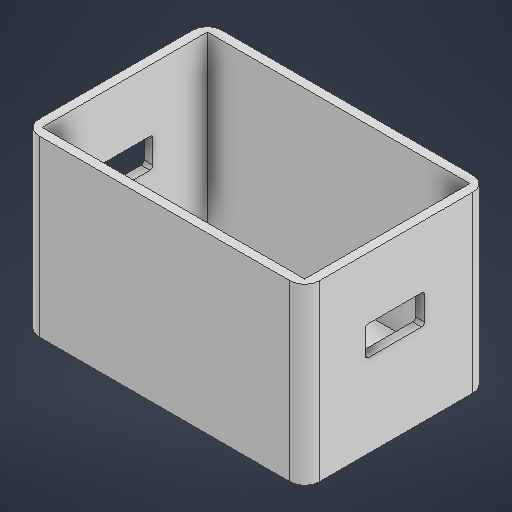
# Autodesk Inventor part: bottom
Saved by Autodesk Inventor 2026.1 (Build 301233020, 233B)
## iProperties
Created: 2025-11-06
Part Number: bottom
Material: Generisch
Document SubType Name: Modeling
Designer: sarae
Density: 1 g/cm^3
Appearance: Vorgabe
Author: sarae
Autodesk Inventor part; units mm, degrees
ref_plane "YZ Plane" through (0, 0, 0) normal (1, 0, 0) x (0, 1, 0)
ref_plane "XZ Plane" through (0, 0, 0) normal (0, 1, 0) x (-1, 0, 0)
ref_plane "XY Plane" through (0, 0, 0) normal (0, 0, 1) x (1, 0, 0)
sketch "Skizze1" plane through (0, 0, 0) normal (0, 0, 1) x (1, 0, 0)
  line L0 (-4.424, 3.089) -> (90.576, 3.089)
  line L1 (90.576, 3.089) -> (90.576, -58.911)
  line L2 (90.576, -58.911) -> (-4.424, -58.911)
  line L3 (-4.424, -58.911) -> (-4.424, 3.089)
  line L4 (-1.424, 0.089) -> (87.576, 0.089)
  line L5 (87.576, 0.089) -> (87.576, -55.911)
  line L6 (87.576, -55.911) -> (-1.424, -55.911)
  line L7 (-1.424, -55.911) -> (-1.424, 0.089)
  point P0 (0, 0)
  dimension "d0" = 95
  dimension "d1" = 62
  dimension "d2" = 89
  dimension "d3" = 56
  dimension "d4" = 3
  dimension "d5" = 3
  constraints: 16 end point, 4 parallel, 2 horizontal, 2 perpendicular
  measures "d0" distance of L1.end L2.end
  measures "d1" distance of L0.end L1.end
  measures "d2" distance of L5.end L6.end
  measures "d3" distance of L4.end L5.end
  measures "d4" distance between parallel lines of L0 L4
  measures "d5" distance between parallel lines of L7 L3
extrude "Extrusion1" add sketch "Skizze1" along normal blind 3 contours L0 L1 L2 L3 | L4 L5 L6 L7
sketch "Skizze2" plane through (0, 0, 3) normal (0, 0, 1) x (1, 0, 0)
  line L0 (90.576, 3.089) -> (-4.424, 3.089) projected
  line L1 (90.576, -58.911) -> (90.576, 3.089) projected
  line L2 (-4.424, 3.089) -> (90.576, 3.089)
  line L3 (90.576, 3.089) -> (90.576, -58.911)
  line L4 (90.576, -58.911) -> (-4.424, -58.911)
  line L5 (-4.424, -58.911) -> (-4.424, 3.089)
  line L6 (-4.424, 3.089) -> (90.576, 3.089)
  line L7 (90.576, 3.089) -> (90.576, -58.911)
  line L8 (90.576, -58.911) -> (-4.424, -58.911)
  line L9 (-4.424, -58.911) -> (-4.424, 3.089)
  line L10 (-1.424, 0.089) -> (87.576, 0.089)
  line L11 (87.576, 0.089) -> (87.576, -55.911)
  line L12 (87.576, -55.911) -> (-1.424, -55.911)
  line L13 (-1.424, -55.911) -> (-1.424, 0.089)
  point P0 (0, 0)
  point P1 (-4.124, -58.911)
  point P2 (4.776, -58.911)
  dimension "d8" = 89
  dimension "d9" = 56
  dimension "d10" = 3
  dimension "d11" = 3
  constraints: 24 end point, 6 parallel, 3 horizontal, 3 perpendicular
  measures "d8" distance of L11.end L12.end
  measures "d9" distance of L10.end L11.end
  measures "d10" distance between parallel lines of L0 L10
  measures "d11" distance between parallel lines of L13 L5
extrude "Extrusion2" add sketch "Skizze2" along normal blind 56
fillet "Rundung1" radius 5 4 edges at (90.576, -58.911, 29.5) (90.576, 3.089, 29.5) (-4.424, -58.911, 29.5) (-4.424, 3.089, 29.5)
sketch "Skizze3" plane through (90.576, -53.911, 0) normal (1, 0, 0) x (0, 0, -1)
  line L0 (-38.1185, 15.5893) -> (-28.1185, 15.5893)
  line L1 (-28.1185, 15.5893) -> (-28.1185, 35.5893)
  line L2 (-28.1185, 35.5893) -> (-38.1185, 35.5893)
  line L3 (-38.1185, 35.5893) -> (-38.1185, 15.5893)
  point P0 (0, 53.911)
  dimension "d15" = 10
  dimension "d16" = 20
  constraints: 8 end point, 2 parallel, 1 horizontal, 1 perpendicular
  measures "d15" distance of L2.end L1.end
  measures "d16" distance of L1.end L0.end
extrude "Extrusion3" cut sketch "Skizze3" against normal blind 100
fillet "Rundung2" radius 1 8 edges at (89.076, -38.3217, 28.1185) (89.076, -18.3217, 28.1185) (89.076, -18.3217, 38.1185) (89.076, -38.3217, 38.1185) (-2.924, -38.3217, 28.1185) (-2.924, -18.3217, 28.1185) (-2.924, -18.3217, 38.1185) (-2.924, -38.3217, 38.1185)
equation "\"d12\" = d9"
